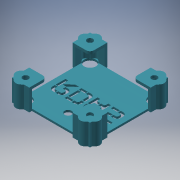
# Autodesk Inventor part: BaseBoardsMiddle_Top
Saved by Autodesk Inventor 2016 (Build 200138000, 138)
## iProperties
Created: 2015-03-29
Part Number: BaseBoardsMiddle_Top
Material: PC/ABS Plastic
Document SubType Name: Modeling
Designer: Erin
Density: 0.357273 g/cm^3
Appearance: Cadet Blue
Mass: 3.14413 g
Surface Area: 66.4965 cm^2
Volume: 5.71659 cm^3
Author: Erin
Autodesk Inventor part; units mm, degrees
ref_plane "YZ Plane" through (0, 0, 0) normal (1, 0, 0) x (0, 1, 0)
ref_plane "XZ Plane" through (0, 0, 0) normal (0, 1, 0) x (-1, 0, 0)
ref_plane "XY Plane" through (0, 0, 0) normal (0, 0, 1) x (1, 0, 0)
sketch "Sketch1" plane through (0, 0, 0) normal (0, 0, 1) x (1, 0, 0)
  line L0 (-48, 48) -> (48, 48)
  line L1 (48, 48) -> (48, -48)
  line L2 (48, -48) -> (-48, -48)
  line L3 (-48, -48) -> (-48, 48)
  line L4 (38, 38) -> (-38, 38)
  line L5 (-38, 38) -> (-38, -38)
  line L6 (-38, -38) -> (38, -38)
  line L7 (38, -38) -> (38, 38)
  line L8 (0, 152.7233) -> (0, -72.1628) construction
  line L9 (-77.8847, 0) -> (88.8171, 0) construction
  line L10 (-48, 43) -> (48, 43) construction
  line L11 (-43, 48) -> (-43, -48) construction
  line L12 (-48, -43) -> (48, -43) construction
  circle A0 centre (-43, 25) radius 2.25
  circle A1 centre (-43, -25) radius 2.25
  circle A2 centre (-43, -43) radius 2.25
  circle A3 centre (-43, 43) radius 2.25
  line L13 (-48, 30) -> (48, 30) construction
  line L14 (-48, -30) -> (48, -30) construction
  line L15 (-50, 31) -> (-36, 31)
  line L16 (-36, 31) -> (-36, -31)
  line L17 (-36, -31) -> (-50, -31)
  line L18 (-50, -31) -> (-50, 31)
  point P0 (0, 0)
  point P1 (0, 48)
  point P2 (48, 0)
  dimension "d0" = 96
  dimension "d1" = 96
  dimension "d2" = 10
  dimension "d5" = 5
  dimension "d11" = 5
  dimension "d14" = 5
  dimension "d31" = 4.5
  dimension "d32" = 4.5
  dimension "d61" = 4.5
  dimension "d62" = 4.5
  dimension "d65" = 30
  dimension "d66" = 30
  dimension "d67" = 5
  dimension "d68" = 5
  dimension "d74" = 1
  dimension "d75" = 1
  dimension "d76" = 2
  dimension "d77" = 2
  constraints: 38 end point, 16 point on line, 9 perpendicular, 7 parallel, 4 centre point, 3 horizontal, 2 midpoint, 1 horizontal alignment, 1 vertical, 1 vertical alignment, 3 other
  measures "d0" distance of L1.end L2.end
  measures "d1" distance of L0.end L1.end
  measures "d2" distance between parallel lines of L4 L0
  measures "d5" distance between parallel lines of L10 L0
  measures "d11" distance between parallel lines of L11 L3
  measures "d14" distance between parallel lines of L12 L2
  measures "d31" diameter of A0
  measures "d32" diameter of A1
  measures "d61" diameter of A2
  measures "d62" diameter of A3
  measures "d65" distance between parallel lines of L13 L9
  measures "d66" distance between parallel lines of L14 L9
  measures "d67" distance from line of A1.centre L14
  measures "d68" distance from line of A0.centre L13
  measures "d74" distance between parallel lines of L13 L15
  measures "d75" distance between parallel lines of L17 L14
  measures "d76" distance between parallel lines of L3 L18
  measures "d77" distance between parallel lines of L16 L5
sketch "Sketch3" plane through (0, 0, 0) normal (0, 0, 1) x (1, 0, 0)
  circle A0 centre (-43, 43) radius 2.25 projected
  circle A1 centre (-43, -43) radius 2.25 projected
  line L0 (48, -48) -> (-48, -48) projected
  line L1 (-48, -48) -> (-48, 48) projected
  line L2 (-38, -38) -> (38, -38) projected
  line L3 (-38, 38) -> (-38, -38) projected
  line L4 (38, 38) -> (-38, 38) projected
  line L5 (-48, 48) -> (48, 48) projected
  line L6 (0, 62.8599) -> (0, -69.2948) construction
  line L7 (-75.2692, 0) -> (82.2152, 0) construction
  line L8 (-28, 28) -> (28, 28)
  line L9 (28, 28) -> (28, -28)
  line L10 (28, -28) -> (-28, -28)
  line L11 (-28, -28) -> (-28, 28)
  line L12 (38, -38) -> (38, 38) projected
  line L13 (48, 48) -> (48, -48) projected
  line L14 (-31.0678, -24.7038) -> (24.7038, 31.0678)
  line L15 (24.7038, 31.0678) -> (31.0678, 24.7038)
  line L16 (31.0678, 24.7038) -> (-24.7038, -31.0678)
  line L17 (-24.7038, -31.0678) -> (-31.0678, -24.7038)
  line L18 (-37.8254, -37.8254) -> (27.8858, 27.8858) construction
  line L19 (-3.182, 3.182) -> (3.182, -3.182) construction
  line L20 (-48, -48) -> (-29.3, -48)
  line L21 (-29.3, -48) -> (-29.3, -29.3)
  line L22 (-29.3, -29.3) -> (-48, -29.3)
  line L23 (-48, -29.3) -> (-48, -48)
  line L24 (-35.664, -29.3) -> (-25.0574, -18.6934)
  line L25 (-25.0574, -18.6934) -> (-18.6934, -25.0574)
  line L26 (-18.6934, -25.0574) -> (-29.3, -35.664)
  line L27 (-29.3, -35.664) -> (-35.664, -29.3)
  line L28 (-32.482, -32.482) -> (-21.8754, -21.8754) construction
  line L29 (-30.3607, -23.9967) -> (-23.9967, -30.3607) construction
  circle A2 centre (-24.7038, -24.7038) radius 2.25
  line L30 (-21, 21) -> (21, 21)
  line L31 (21, 21) -> (21, -21)
  line L32 (21, -21) -> (-21, -21)
  line L33 (-21, -21) -> (-21, 21)
  point P0 (0, 0)
  point P1 (0, 0)
  point P2 (0, 21)
  point P3 (0, 28)
  point P4 (21, 0)
  point P5 (28, 0)
  dimension "d80" = 9
  dimension "d81" = 18.7
  dimension "d83" = 10
  dimension "d84" = 10
  dimension "d85" = 10
  dimension "d86" = 10
  dimension "d98" = 15
  dimension "d99" = 9
  dimension "d100" = 4.5
  dimension "d101" = 4
  dimension "d102" = 1
  dimension "d108" = 18.7
  dimension "d113" = 42
  dimension "d114" = 42
  constraints: 52 end point, 12 midpoint, 10 parallel, 5 horizontal, 5 perpendicular, 5 point on line, 2 vertical, 1 centre point, 1 coincident, 1 horizontal alignment, 1 vertical alignment
  measures "d80" distance of L14.end L15.end
  measures "d81" distance of L21.end L22.end
  measures "d83" distance between parallel lines of L3 L11
  measures "d84" distance between parallel lines of L4 L8
  measures "d85" distance between parallel lines of L12 L9
  measures "d86" distance between parallel lines of L2 L10
  measures "d98" distance of L25.end L26.end
  measures "d99" distance of L24.end L25.end
  measures "d100" diameter of A2
  measures "d101" distance from line of A2.centre L25
  measures "d102" distance between parallel lines of L29 L17
  measures "d108" distance of L20.end L21.end
  measures "d113" distance of L30.start L30.end
  measures "d114" distance of L30.end L31.end
extrude "Extrusion7" add sketch "Sketch3" along normal blind 1.5 contours L16 L32 L31 L9 L10 | L10 L17 L11 L14 L25 L16 | L10 L11 L17 | L25 L14 L33 L32 L16 | L11 L8 L14 L30 L33 | L16 L31 L30 L14 L8 L15 L9 | L32 L33 L14 L30 L31 L16 | L16 L31 L32 | L15 L8 L9 | L33 L30 L14 | A2
extrude "Extrusion9" add sketch "Sketch3" along normal blind 1.5 contours L17 L10 L16 | L10 L17 L11 L14 L25 L16 | L14 L11 L17 | L25 L14 L33 L32 L16 | L16 L31 L30 L14 L8 L15 L9 | L9 L15 L16 | L32 L33 L14 L30 L31 L16 | L14 L15 L8 | A2
mirror "Mirror6" about plane through (0, 0, 0) normal (1, 0, 0) of "Extrusion9"
extrude "Extrusion10" cut sketch "Sketch3" along normal blind 10 contours A2
pattern_circular "Circular Pattern3" count 4 over 360 about axis through (0, 0, -10) along (0, 0, 1) of "Extrusion10"
fillet "Fillet2" radius 2 2 edges at (-24.7038, -31.0678, 0.75) (-31.0678, -24.7038, 0.75)
pattern_circular "Circular Pattern4" count 4 over 360 about axis through (0, 0, -10) along (0, 0, 1) of "Fillet2"
sketch "Sketch4" plane through (0, 0, 1.5) normal (0, 0, 1) x (1, 0, 0)
  arc A0 (-23.2896, 29.6536) -> (-26.118, 29.6536) centre (-24.7038, 28.2393) ccw projected
  line L0 (-27.7716, 28) -> (-26.118, 29.6536) projected
  line L1 (-27.7716, 28) -> (-28, 28) projected
  line L2 (-28, 28) -> (-28, 27.7716) projected
  line L3 (-29.6536, 26.118) -> (-28, 27.7716) projected
  arc A1 (-29.6536, 26.118) -> (-29.6536, 23.2896) centre (-28.2393, 24.7038) ccw projected
  line L4 (-28, 21.636) -> (-29.6536, 23.2896) projected
  line L5 (-28, 21.636) -> (-28, -21.636) projected
  line L6 (-28, -21.636) -> (-29.6536, -23.2896) projected
  arc A2 (-29.6536, -23.2896) -> (-29.6536, -26.118) centre (-28.2393, -24.7038) ccw projected
  line L7 (-29.6536, -26.118) -> (-28, -27.7716) projected
  line L8 (-28, -27.7716) -> (-28, -28) projected
  line L9 (-28, -28) -> (-27.7716, -28) projected
  line L10 (-27.7716, -28) -> (-26.118, -29.6536) projected
  arc A3 (-26.118, -29.6536) -> (-23.2896, -29.6536) centre (-24.7038, -28.2393) ccw projected
  line L11 (-23.2896, -29.6536) -> (-21.636, -28) projected
  line L12 (-21.636, -28) -> (21.636, -28) projected
  line L13 (23.2896, -29.6536) -> (21.636, -28) projected
  arc A4 (23.2896, -29.6536) -> (26.118, -29.6536) centre (24.7038, -28.2393) ccw projected
  line L14 (27.7716, -28) -> (26.118, -29.6536) projected
  line L15 (27.7716, -28) -> (28, -28) projected
  line L16 (28, -28) -> (28, -27.7716) projected
  line L17 (29.6536, -26.118) -> (28, -27.7716) projected
  arc A5 (29.6536, -26.118) -> (29.6536, -23.2896) centre (28.2393, -24.7038) ccw projected
  line L18 (28, -21.636) -> (29.6536, -23.2896) projected
  line L19 (28, -21.636) -> (28, 21.636) projected
  line L20 (28, 21.636) -> (29.6536, 23.2896) projected
  arc A6 (29.6536, 23.2896) -> (29.6536, 26.118) centre (28.2393, 24.7038) ccw projected
  line L21 (29.6536, 26.118) -> (28, 27.7716) projected
  line L22 (28, 27.7716) -> (28, 28) projected
  line L23 (28, 28) -> (27.7716, 28) projected
  line L24 (27.7716, 28) -> (26.118, 29.6536) projected
  arc A7 (26.118, 29.6536) -> (23.2896, 29.6536) centre (24.7038, 28.2393) ccw projected
  line L25 (23.2896, 29.6536) -> (21.636, 28) projected
  line L26 (21.636, 28) -> (-21.636, 28) projected
  line L27 (-23.2896, 29.6536) -> (-21.636, 28) projected
  circle A8 centre (-24.7038, 24.7038) radius 2.25 projected
  circle A9 centre (24.7038, 24.7038) radius 2.25 projected
  circle A10 centre (24.7038, -24.7038) radius 2.25 projected
  circle A11 centre (-24.7038, -24.7038) radius 2.25 projected
  line L28 (-20.8076, 30) -> (-16.636, 30)
  line L29 (20.8076, 30) -> (21.8754, 31.0678)
  arc A12 (27.5322, 31.0678) -> (21.8754, 31.0678) centre (24.7038, 28.2393) ccw
  line L30 (27.5322, 31.0678) -> (28.6, 30)
  line L31 (28.6, 30) -> (30, 30)
  line L32 (30, 30) -> (30, 28.6)
  line L33 (30, 28.6) -> (31.0678, 27.5322)
  arc A13 (31.0678, 21.8754) -> (31.0678, 27.5322) centre (28.2393, 24.7038) ccw
  line L34 (31.0678, 21.8754) -> (30, 20.8076)
  line L35 (30, 20.8076) -> (30, -20.8076)
  line L36 (30, -20.8076) -> (31.0678, -21.8754)
  arc A14 (31.0678, -27.5322) -> (31.0678, -21.8754) centre (28.2393, -24.7038) ccw
  line L37 (31.0678, -27.5322) -> (30, -28.6)
  line L38 (30, -28.6) -> (30, -30)
  line L39 (30, -30) -> (28.6, -30)
  line L40 (28.6, -30) -> (27.5322, -31.0678)
  arc A15 (21.8754, -31.0678) -> (27.5322, -31.0678) centre (24.7038, -28.2393) ccw
  line L41 (21.8754, -31.0678) -> (20.8076, -30)
  line L42 (20.8076, -30) -> (-20.8076, -30)
  line L43 (-20.8076, -30) -> (-21.8754, -31.0678)
  arc A16 (-27.5322, -31.0678) -> (-21.8754, -31.0678) centre (-24.7038, -28.2393) ccw
  line L44 (-27.5322, -31.0678) -> (-28.6, -30)
  line L45 (-28.6, -30) -> (-30, -30)
  line L46 (-30, -30) -> (-30, -28.6)
  line L47 (-30, -28.6) -> (-31.0678, -27.5322)
  arc A17 (-31.0678, -21.8754) -> (-31.0678, -27.5322) centre (-28.2393, -24.7038) ccw
  line L48 (-31.0678, -21.8754) -> (-30, -20.8076)
  line L49 (-30, 16.636) -> (-30, 20.8076)
  line L50 (-30, 20.8076) -> (-31.0678, 21.8754)
  arc A18 (-31.0678, 27.5322) -> (-31.0678, 21.8754) centre (-28.2393, 24.7038) ccw
  line L51 (-31.0678, 27.5322) -> (-30, 28.6)
  line L52 (-30, 28.6) -> (-30, 30)
  line L53 (-30, 30) -> (-28.6, 30)
  line L54 (-28.6, 30) -> (-27.5322, 31.0678)
  arc A19 (-21.8754, 31.0678) -> (-27.5322, 31.0678) centre (-24.7038, 28.2393) ccw
  line L55 (-21.8754, 31.0678) -> (-20.8076, 30)
  line L56 (-30, 16.636) -> (-28, 16.636)
  line L57 (-16.636, 30) -> (-16.636, 28)
  line L58 (-21.636, 28) -> (21.636, 28) projected
  line L59 (-28, 16.636) -> (-16.636, 16.636)
  line L60 (-16.636, 16.636) -> (-16.636, 28)
  circle A20 centre (-24.7038, 24.7038) radius 2.25 projected
  circle A21 centre (-24.7038, 24.7038) radius 4.5029
  point P0 (0, 0)
  dimension "d118" = 2
  dimension "d119" = 5
  dimension "d120" = 5
  constraints: 64 end point, 16 point on circle, 8 centre point, 2 perpendicular, 2 point on line, 1 coincident, 1 collinear, 1 horizontal, 35 other
  measures "d118" distance between parallel lines of L28 L26
  measures "d119" distance from line of L26.end L57
  measures "d120" distance from line of L4.start L56
extrude "Extrusion12" add sketch "Sketch4" along normal blind 15 contours L27 A21 L0 A0 | A0 L0 L1 L2 L3 A1 L4 L5 L56 L49 L50 A18 L51 L52 L53 L54 A19 L55 L28 L57 L26 L27 | L26 L60 L59 L5 A21 | A21 | A21 L2 L1 | A21 L4 A1 L3
extrude "Extrusion13" cut sketch "Sketch4" along normal blind 13 contours L27 A21 L0 A0 | L26 L60 L59 L5 A21 | A21 | A21 L2 L1 | A21 L4 A1 L3
fillet "Fillet4" radius 3 1 edges at (-16.636, 16.636, 15.5)
extrude "Extrusion14" cut sketch "Sketch4" against normal blind 3 contours A21
extrude "Extrusion15" add sketch "Sketch4" against normal blind 1.5 contours A0 L0 L1 L2 L3 A1 L4 L5 L56 L49 L50 A18 L51 L52 L53 L54 A19 L55 L28 L57 L26 L27
pattern_circular "Circular Pattern5" count 4 over 360 about axis through (0, 0, -10) along (0, 0, 1) of "Extrusion12", "Extrusion13", "Fillet4", "Extrusion14", "Extrusion15"
sketch "Sketch6" plane through (0, 0, 0) normal (0, 0, -1) x (-1, 0, 0)
  line L0 (24.5493, -8.2866) -> (-13.3532, -8.2866) construction
  line L1 (-13.3532, -8.2866) -> (-13.3532, 1.7134) construction
  line L2 (-13.3532, 1.7134) -> (24.5493, 1.7134) construction
  line L3 (24.5493, 1.7134) -> (24.5493, -8.2866) construction
  circle A0 centre (0, -16.7986) radius 2.7
  spline S0 degree 2 poles (15.3106, -3.8357) (15.3106, -3.4106) (15.896, -2.8091) (16.3371, -2.8091) knots 0 0 0 1 2 2 2
  line L4 (16.3371, -2.8091) -> (18.0453, -2.8091)
  line L5 (18.0453, -2.8091) -> (18.0453, -0.7561)
  line L6 (18.0453, -0.7561) -> (16.3371, -0.7561)
  spline S1 degree 2 poles (16.3371, -0.7561) (15.7035, -0.7561) (14.5727, -1.2373) (13.7387, -2.0713) (13.2575, -3.2021) (13.2575, -3.8357) knots 0 0 0 1 2 3 4 4 4
  line L7 (13.2575, -3.8357) -> (13.2575, -5.207)
  spline S2 degree 2 poles (13.2575, -5.207) (13.2575, -5.8406) (13.7387, -6.9714) (14.5727, -7.8054) (15.7035, -8.2866) (16.3371, -8.2866) knots 0 0 0 1 2 3 4 4 4
  line L8 (16.3371, -8.2866) -> (18.0453, -8.2866)
  line L9 (18.0453, -8.2866) -> (18.0453, -6.2336)
  line L10 (18.0453, -6.2336) -> (16.3371, -6.2336)
  spline S3 degree 2 poles (16.3371, -6.2336) (15.896, -6.2336) (15.3106, -5.6321) (15.3106, -5.207) knots 0 0 0 1 2 2 2
  line L11 (15.3106, -5.207) -> (15.3106, -3.8357)
  line L12 (21.4697, 4.7134) -> (23.5228, 4.7134)
  line L13 (23.5228, 4.7134) -> (23.5228, -2.8091)
  line L14 (23.5228, -2.8091) -> (21.4697, -2.8091)
  line L15 (21.4697, -2.8091) -> (21.4697, 4.7134)
  line L16 (13.2575, 4.7134) -> (13.2575, 4.2883)
  line L17 (13.2575, 4.2883) -> (18.1656, -0.0744)
  line L18 (18.1656, -0.0744) -> (20.788, -0.0744)
  line L19 (20.788, -0.0744) -> (20.788, 0.3506)
  line L20 (20.788, 0.3506) -> (15.8559, 4.7134)
  line L21 (15.8559, 4.7134) -> (13.2575, 4.7134)
  spline S4 degree 2 poles (20.4432, -6.2336) (20.8682, -6.2336) (21.4697, -5.6321) (21.4697, -5.207) knots 0 0 0 1 2 2 2
  line L22 (21.4697, -5.207) -> (21.4697, -3.4988)
  line L23 (21.4697, -3.4988) -> (23.5228, -3.4988)
  line L24 (23.5228, -3.4988) -> (23.5228, -5.207)
  spline S5 degree 2 poles (23.5228, -5.207) (23.5228, -5.8406) (23.0416, -6.9714) (22.2075, -7.8054) (21.0768, -8.2866) (20.4432, -8.2866) knots 0 0 0 1 2 3 4 4 4
  line L25 (20.4432, -8.2866) -> (18.735, -8.2866)
  line L26 (18.735, -8.2866) -> (18.735, -6.2336)
  line L27 (18.735, -6.2336) -> (20.4432, -6.2336)
  spline S6 degree 2 poles (4.0188, 2.6603) (3.5777, 2.6603) (2.9922, 2.0588) (2.9922, 1.6338) knots 0 0 0 1 2 2 2
  line L28 (2.9922, 1.6338) -> (2.9922, -2.8172)
  line L29 (2.9922, -2.8172) -> (0.9392, -2.8172)
  line L30 (0.9392, -2.8172) -> (0.9392, 1.6338)
  spline S7 degree 2 poles (0.9392, 1.6338) (0.9392, 2.2674) (1.4204, 3.3981) (2.2544, 4.2322) (3.3852, 4.7134) (4.0188, 4.7134) knots 0 0 0 1 2 3 4 4 4
  line L31 (4.0188, 4.7134) -> (5.727, 4.7134)
  line L32 (5.727, 4.7134) -> (5.727, 2.6603)
  line L33 (5.727, 2.6603) -> (4.0188, 2.6603)
  line L34 (11.2045, -5.5519) -> (9.1514, -5.5519)
  line L35 (9.1514, -5.5519) -> (9.1514, 1.9786)
  line L36 (9.1514, 1.9786) -> (11.2045, 1.9786)
  line L37 (11.2045, 1.9786) -> (11.2045, -5.5519)
  spline S8 degree 2 poles (2.9922, -5.207) (2.9922, -5.6321) (3.5777, -6.2336) (4.0188, -6.2336) knots 0 0 0 1 2 2 2
  line L38 (4.0188, -6.2336) -> (5.727, -6.2336)
  line L39 (5.727, -6.2336) -> (5.727, -8.2866)
  line L40 (5.727, -8.2866) -> (4.0188, -8.2866)
  spline S9 degree 2 poles (4.0188, -8.2866) (3.3852, -8.2866) (2.2544, -7.8054) (1.4204, -6.9714) (0.9392, -5.8406) (0.9392, -5.207) knots 0 0 0 1 2 3 4 4 4
  line L41 (0.9392, -5.207) -> (0.9392, -3.4988)
  line L42 (0.9392, -3.4988) -> (2.9922, -3.4988)
  line L43 (2.9922, -3.4988) -> (2.9922, -5.207)
  line L44 (6.4167, 2.6603) -> (6.4167, 4.7134)
  line L45 (6.4167, 4.7134) -> (11.2045, 4.7134)
  line L46 (11.2045, 4.7134) -> (11.2045, 2.6603)
  line L47 (11.2045, 2.6603) -> (6.4167, 2.6603)
  line L48 (6.4167, -8.2866) -> (6.4167, -6.2336)
  line L49 (6.4167, -6.2336) -> (11.2045, -6.2336)
  line L50 (11.2045, -6.2336) -> (11.2045, -8.2866)
  line L51 (11.2045, -8.2866) -> (6.4167, -8.2866)
  line L52 (-5.9017, -0.0744) -> (-5.9017, 1.9786)
  line L53 (-5.9017, 1.9786) -> (-4.1935, 1.9786)
  spline S10 degree 2 poles (-4.1935, 1.9786) (-3.7684, 1.9786) (-3.1669, 2.5801) (-3.1669, 3.0052) knots 0 0 0 1 2 2 2
  line L54 (-3.1669, 3.0052) -> (-3.1669, 4.7134)
  line L55 (-3.1669, 4.7134) -> (-1.1139, 4.7134)
  line L56 (-1.1139, 4.7134) -> (-1.1139, -2.8091)
  line L57 (-1.1139, -2.8091) -> (-3.1669, -2.8091)
  line L58 (-3.1669, -2.8091) -> (-3.1669, -1.1009)
  spline S11 degree 2 poles (-3.1669, -1.1009) (-3.1669, -0.6759) (-3.7684, -0.0744) (-4.1935, -0.0744) knots 0 0 0 1 2 2 2
  line L59 (-4.1935, -0.0744) -> (-5.9017, -0.0744)
  line L60 (-6.5914, 1.9786) -> (-6.5914, -0.0744)
  line L61 (-6.5914, -0.0744) -> (-8.2996, -0.0744)
  spline S12 degree 2 poles (-8.2996, -0.0744) (-8.7406, -0.0744) (-9.3261, -0.6759) (-9.3261, -1.1009) knots 0 0 0 1 2 2 2
  line L62 (-9.3261, -1.1009) -> (-9.3261, -2.8091)
  line L63 (-9.3261, -2.8091) -> (-11.3791, -2.8091)
  line L64 (-11.3791, -2.8091) -> (-11.3791, 4.7134)
  line L65 (-11.3791, 4.7134) -> (-9.3261, 4.7134)
  line L66 (-9.3261, 4.7134) -> (-9.3261, 3.0052)
  spline S13 degree 2 poles (-9.3261, 3.0052) (-9.3261, 2.5801) (-8.7406, 1.9786) (-8.2996, 1.9786) knots 0 0 0 1 2 2 2
  line L67 (-8.2996, 1.9786) -> (-6.5914, 1.9786)
  line L68 (-3.1669, -3.4988) -> (-1.1139, -3.4988)
  line L69 (-1.1139, -3.4988) -> (-1.1139, -5.207)
  spline S14 degree 2 poles (-1.1139, -5.207) (-1.1139, -5.8406) (-1.5951, -6.9714) (-2.4291, -7.8054) (-3.5599, -8.2866) (-4.1935, -8.2866) knots 0 0 0 1 2 3 4 4 4
  line L70 (-4.1935, -8.2866) -> (-5.9017, -8.2866)
  line L71 (-5.9017, -8.2866) -> (-5.9017, -6.2336)
  line L72 (-5.9017, -6.2336) -> (-4.1935, -6.2336)
  spline S15 degree 2 poles (-4.1935, -6.2336) (-3.7684, -6.2336) (-3.1669, -5.6321) (-3.1669, -5.207) knots 0 0 0 1 2 2 2
  line L73 (-3.1669, -5.207) -> (-3.1669, -3.4988)
  line L74 (-6.5914, -6.2336) -> (-6.5914, -8.2866)
  line L75 (-6.5914, -8.2866) -> (-8.2996, -8.2866)
  spline S16 degree 2 poles (-8.2996, -8.2866) (-8.9331, -8.2866) (-10.0639, -7.8054) (-10.898, -6.9714) (-11.3791, -5.8406) (-11.3791, -5.207) knots 0 0 0 1 2 3 4 4 4
  line L76 (-11.3791, -5.207) -> (-11.3791, -3.4988)
  line L77 (-11.3791, -3.4988) -> (-9.3261, -3.4988)
  line L78 (-9.3261, -3.4988) -> (-9.3261, -5.207)
  spline S17 degree 2 poles (-9.3261, -5.207) (-9.3261, -5.6321) (-8.7406, -6.2336) (-8.2996, -6.2336) knots 0 0 0 1 2 2 2
  line L79 (-8.2996, -6.2336) -> (-6.5914, -6.2336)
  spline S18 degree 2 poles (-21.6444, 1.6338) (-21.6444, 2.0588) (-21.059, 2.6603) (-20.6179, 2.6603) knots 0 0 0 1 2 2 2
  line L80 (-20.6179, 2.6603) -> (-18.9097, 2.6603)
  line L81 (-18.9097, 2.6603) -> (-18.9097, 4.7134)
  line L82 (-18.9097, 4.7134) -> (-20.6179, 4.7134)
  spline S19 degree 2 poles (-20.6179, 4.7134) (-21.2514, 4.7134) (-22.3822, 4.2322) (-23.2163, 3.3981) (-23.6975, 2.2674) (-23.6975, 1.6338) knots 0 0 0 1 2 3 4 4 4
  line L83 (-23.6975, 1.6338) -> (-23.6975, 0.2624)
  spline S20 degree 2 poles (-23.6975, 0.2624) (-23.6975, -0.3711) (-23.2163, -1.5019) (-22.3822, -2.336) (-21.2514, -2.8172) (-20.6179, -2.8172) knots 0 0 0 1 2 3 4 4 4
  line L84 (-20.6179, -2.8172) -> (-18.9097, -2.8172)
  line L85 (-18.9097, -2.8172) -> (-18.9097, -0.7641)
  line L86 (-18.9097, -0.7641) -> (-20.6179, -0.7641)
  spline S21 degree 2 poles (-20.6179, -0.7641) (-21.059, -0.7641) (-21.6444, -0.1626) (-21.6444, 0.2624) knots 0 0 0 1 2 2 2
  line L87 (-21.6444, 0.2624) -> (-21.6444, 1.6338)
  spline S22 degree 2 poles (-15.4852, -5.207) (-15.4852, -5.6321) (-16.0867, -6.2336) (-16.5118, -6.2336) knots 0 0 0 1 2 2 2
  line L88 (-16.5118, -6.2336) -> (-18.22, -6.2336)
  line L89 (-18.22, -6.2336) -> (-18.22, -8.2866)
  line L90 (-18.22, -8.2866) -> (-16.5118, -8.2866)
  spline S23 degree 2 poles (-16.5118, -8.2866) (-15.8782, -8.2866) (-14.7474, -7.8054) (-13.9134, -6.9714) (-13.4322, -5.8406) (-13.4322, -5.207) knots 0 0 0 1 2 3 4 4 4
  line L91 (-13.4322, -5.207) -> (-13.4322, -3.8437)
  spline S24 degree 2 poles (-13.4322, -3.8437) (-13.4322, -3.2101) (-13.9134, -2.0793) (-14.7474, -1.2453) (-15.8782, -0.7641) (-16.5118, -0.7641) knots 0 0 0 1 2 3 4 4 4
  line L92 (-16.5118, -0.7641) -> (-18.22, -0.7641)
  line L93 (-18.22, -0.7641) -> (-18.22, -2.8172)
  line L94 (-18.22, -2.8172) -> (-16.5118, -2.8172)
  spline S25 degree 2 poles (-16.5118, -2.8172) (-16.0867, -2.8172) (-15.4852, -3.4186) (-15.4852, -3.8437) knots 0 0 0 1 2 2 2
  line L95 (-15.4852, -3.8437) -> (-15.4852, -5.207)
  line L96 (-13.4322, 4.7134) -> (-13.4322, 2.6603)
  line L97 (-13.4322, 2.6603) -> (-18.22, 2.6603)
  line L98 (-18.22, 2.6603) -> (-18.22, 4.7134)
  line L99 (-18.22, 4.7134) -> (-13.4322, 4.7134)
  line L100 (-18.9097, -6.2336) -> (-18.9097, -8.2866)
  line L101 (-18.9097, -8.2866) -> (-23.6975, -8.2866)
  line L102 (-23.6975, -8.2866) -> (-23.6975, -6.2336)
  line L103 (-23.6975, -6.2336) -> (-18.9097, -6.2336)
  point P0 (0, 0)
  dimension "d133" = 5.4
  constraints: 1 centre point, 2 other
  measures "d133" diameter of A0
extrude "Extrusion16" cut sketch "Sketch6" against normal blind 3
equation "\"d31\" = screw"
equation "\"d32\" = screw"
equation "\"d61\" = screw"
equation "\"d62\" = screw"
equation "\"screw\" = 4.5"
body "Solid2"
